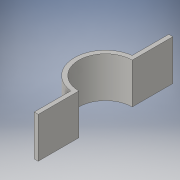
# Autodesk Inventor part: Attachy-thing
Saved by Autodesk Inventor 2016 (Build 200138000, 138)
## iProperties
Created: 2017-01-30
Part Number: Attachy-thing
Material: Generic
Document SubType Name: Modeling
Designer: student1
Density: 1 g/cm^3
Appearance: Default
Author: student1
Autodesk Inventor part; units mm, degrees
ref_plane "YZ Plane" through (0, 0, 0) normal (1, 0, 0) x (0, 1, 0)
ref_plane "XZ Plane" through (0, 0, 0) normal (0, 1, 0) x (-1, 0, 0)
ref_plane "XY Plane" through (0, 0, 0) normal (0, 0, 1) x (1, 0, 0)
sketch "Sketch1" plane through (0, 0, 0) normal (0, 1, 0) x (-1, 0, 0)
  arc A0 (0, -21.6252) -> (0, 11.7758) centre (0, -4.9247) ccw
  line L0 (0, 37.1885) -> (0, 11.7885)
  line L1 (0, -21.6379) -> (0, -47.0379)
  arc A1 (0, -21.6379) -> (0, 11.7885) centre (0, -4.9247) ccw
  line L2 (0, 37.1885) -> (2.54, 37.1885)
  line L3 (0, -47.0379) -> (2.54, -47.0379)
  line L4 (2.54, 37.1885) -> (2.54, 14.3285)
  line L5 (2.54, -47.0379) -> (2.54, -24.1779)
  arc A2 (2.54, -24.1779) -> (2.54, 14.3285) centre (0, -4.9247) ccw
  dimension "d0" = 33.401
  dimension "d1" = 25.4
  dimension "d2" = 25.4
  dimension "d3" = 33.4264
  dimension "d6" = 16.7132
  dimension "d7" = 16.7132
  dimension "d8" = 2.54
  dimension "d9" = 2.54
  dimension "d10" = 19.2532
  dimension "d11" = 19.2532
  constraints: 12 end point, 6 point on circle, 4 vertical, 3 centre point, 2 horizontal, 2 point on line, 1 concentric
  measures "d0" diameter of A0
  measures "d1" distance of L0.start L0.end
  measures "d2" distance of L1.start L1.end
  measures "d3" distance of L1.start L0.end
  measures "d6" distance of L0.end A0.centre
  measures "d7" distance of L1.start A0.centre
  measures "d8" distance of L0.start L2.end
  measures "d9" distance of L1.end L3.end
  measures "d10" vertical distance of L4.end A0.centre
  measures "d11" vertical distance of L5.end A0.centre
extrude "Extrusion1" add sketch "Sketch1" along normal blind 25.4
equation "\"d2\" = d1"
equation "\"d7\" = d6"
equation "\"d9\" = d8"
body "Solid1"
